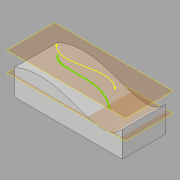
# Autodesk Inventor part: ProjectCurveToSurface
Saved by Autodesk Inventor 2017.2 (Build 212233000, 233)
## iProperties
Created: 2017-03-28
Part Number: ProjectCurveToSurface
Material: Generic
Document SubType Name: Modeling
Designer: alex.fielder
Mass: 1.40668 g
Surface Area: 9.07809 cm^2
Volume: 1.40668 cm^3
Density: 1 g/cm^3
Appearance: Default
Author: alex.fielder
Autodesk Inventor part; units mm, degrees
ref_plane "YZ Plane" through (0, 0, 0) normal (1, 0, 0) x (0, 1, 0)
ref_plane "XY Plane" through (0, 0, 0) normal (0, 0, 1) x (1, 0, 0)
sketch "Sketch1" plane through (0, 0, 0) normal (0, 0, 1) x (1, 0, 0)
  line L0 (-10.8905, 1.433) -> (-10.8905, -4.4626)
  line L1 (-10.8905, -4.4626) -> (13.9201, -4.4626)
  line L2 (13.9201, -4.4626) -> (13.9201, 1.433)
  spline S0 degree 3 poles (13.9201, 1.433) (7.9879, -5.0542) (0.1353, 6.3085) (-10.8905, 1.433) knots 0 0 0 0 1 1 1 1
  point P0 (0, 0)
  point P1 (8.516, -0.5729)
  point P2 (0.737, 1.7197)
  constraints: 6 end point, 2 perpendicular, 1 vertical, 4 other
extrude "Extrusion1" add sketch "Sketch1" along normal mid plane 10
ref_plane "Work Plane1" through (0, 4.5, 0) normal (0, 1, 0) x (-1, 0, 0)
sketch "Sketch2" plane through (0, 4.5, 0) normal (0, 1, 0) x (-1, 0, 0)
  spline S0 degree 3 poles (7.4366, -1.1913) (3.2681, 2.9614) (-3.2799, -3.3624) (-7.8897, 0.6233) knots 0 0 0 0 1 1 1 1
  point P0 (0, 0)
  point P1 (2.878, 0.2606)
  point P2 (-2.789, -0.6953)
  constraints: 4 other
sketch3d "3D Sketch1"
sketch3d "3D Sketch5"
body "Solid1"
